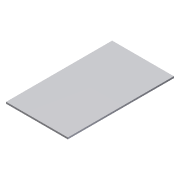
# Autodesk Inventor part: ControlPanel
Saved by Autodesk Inventor 2014 (Build 180170000, 170)
## iProperties
Created: 2015-01-20
Part Number: ControlPanel
Material: Generic
Document SubType Name: Modeling
Designer: Peele
Density: 1 g/cm^3
Appearance: White
Author: Peele
Autodesk Inventor part; units mm, degrees
ref_plane "YZ Plane" through (0, 0, 0) normal (1, 0, 0) x (0, 1, 0)
ref_plane "XZ Plane" through (0, 0, 0) normal (0, 1, 0) x (-1, 0, 0)
ref_plane "XY Plane" through (0, 0, 0) normal (0, 0, 1) x (1, 0, 0)
sketch "Sketch1" plane through (0, 0, 0) normal (0, 0, 1) x (1, 0, 0)
  line L0 (55, -94.5) -> (-55, -94.5)
  line L1 (-55, -94.5) -> (-55, 94.5)
  line L2 (-55, 94.5) -> (55, 94.5)
  line L3 (55, 94.5) -> (55, -94.5)
  line L4 (55, -94.5) -> (-55, 94.5) construction
  line L5 (-55, -94.5) -> (55, 94.5) construction
  point P0 (0, 0)
  dimension "d0" = 189
  dimension "d1" = 110
  constraints: 12 end point, 2 midpoint, 2 parallel, 1 horizontal, 1 perpendicular
  measures "d0" distance of L0.end L1.end
  measures "d1" distance of L0.start L0.end
extrude "Extrusion1" add sketch "Sketch1" along normal blind 3
body "Solid1"
